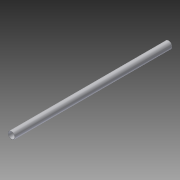
# Autodesk Inventor part: pvcSection
Saved by Autodesk Inventor 2014 (Build 180170000, 170)
## iProperties
Created: 2015-03-27
Part Number: pvcSection
Material: PVC-Piping
Document SubType Name: Modeling
Designer: ddeboer
Mass: 2958.21 g
Surface Area: 10817.7 cm^2
Volume: 2113.01 cm^3
Density: 1.4 g/cm^3
Appearance: Smooth - White
Author: ddeboer
Autodesk Inventor part; units mm, degrees
ref_plane "YZ Plane" through (0, 0, 0) normal (1, 0, 0) x (0, 1, 0)
ref_plane "XZ Plane" through (0, 0, 0) normal (0, 1, 0) x (-1, 0, 0)
ref_plane "XY Plane" through (0, 0, 0) normal (0, 0, 1) x (1, 0, 0)
sketch "Sketch1" plane through (0, 0, 0) normal (0, 0, 1) x (1, 0, 0)
  circle A0 centre (0, 0) radius 30.1625
  circle A1 centre (0, 0) radius 26.2509
  dimension "d0" = 60.325
  dimension "d1" = 3.9116
  constraints: 2 centre point, 1 coincident
  measures "d0" diameter of A0
  measures "d1" radial gap between concentric circles of A1 A0
extrude "Extrusion1" add sketch "Sketch1" along normal blind 1320.8
body "Solid1"
